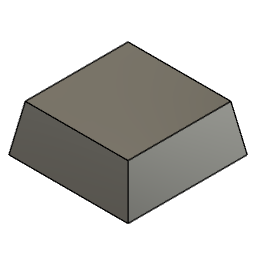
Keycap (Autodesk Fusion 360 design; units mm, degrees)
Autodesk Fusion 360 part; units mm, degrees
sketch "Sketch1" plane through (0, 0, 0) normal (0, 0, 1) x (1, 0, 0)
  line L0 (0, 0) -> (18, 0)
  line L1 (0, 0) -> (0, 7) construction
  line L2 (0, 7) -> (19.3695, 7) construction
  line L3 (18, 0) -> (18, 8.9919) construction
  line L4 (0, 0) -> (1.2343, 7)
  line L5 (0, 0) -> (7.108, 0) construction
  line L6 (18, 0) -> (16.7657, 7)
  line L7 (18, 0) -> (25.108, 0) construction
  line L8 (1.2343, 7) -> (16.7657, 7)
  dimension "d1" = 18
  dimension "d2" = 7
  dimension "d3" = 80
  dimension "d4" = 100
  constraint coincident L0.start L1.start
  constraint horizontal L0
  constraint perpendicular L0 L1
  constraint perpendicular L1 L2
  constraint perpendicular L2 L3
  constraint horizontal L5
  constraint coincident L2 L4.end
  constraint horizontal L7
  constraint coincident L2 L6.end
  measures "d1" distance of L0.start L0.end
  measures "d2" distance of L0.start L1.end
  measures "d3" angle of L4 L5
  measures "d4" angle of L6 L7
extrude "Extrude1" add sketch "Sketch1" along normal blind 18 makes body 1
sketch "Sketch2" plane through (0, 0, 0) normal (1, 0, 0) x (0, 0, -1)
  line L0 (0, 7) -> (0, 0)
  line L1 (0, 0) -> (-18, 0)
  line L2 (-18, 0) -> (-18, 7)
  line L3 (-18, 7) -> (0, 7)
  line L4 (0, 0) -> (-1.2343, 7)
  line L5 (0, 0) -> (7.108, 0) construction
  line L6 (-18, 0) -> (-16.7657, 7)
  line L7 (-18, 0) -> (-10.892, 0) construction
  line L8 (-16.7657, 7) -> (-18, 7)
  line L9 (-18, 7) -> (-18, 0)
  line L10 (-1.2343, 7) -> (0, 7)
  line L11 (0, 7) -> (0, 0)
  dimension "d7" = 100
  dimension "d8" = 80
  constraint horizontal L5
  constraint coincident L0.end L1.start
  constraint coincident L3 L4.end
  constraint horizontal L7
  constraint coincident L1.end L2.start
  constraint coincident L3 L6.end
  constraint coincident L2.end L3.start
  constraint coincident L0.start L3.end
  measures "d7" angle of L4 L5
  measures "d8" angle of L6 L7
extrude "Extrude2" cut sketch "Sketch2" along normal blind 25.5 contours L0 L3 L4 L10 L11 | L2 L3 L6 L8 L9 bodies 1
shell "Shell1" thickness 1.5 removed faces 1 at (6, 0, 6) on bodies 1
sketch "Sketch3" plane through (0, 0, 0) normal (0, 0, 1) x (1, 0, 0)
  line L0 (0, 0) -> (0, 6.75)
  line L1 (3.1, 6.75) -> (3.4, 0)
  line L2 (3.1, 6.75) -> (4.6, 6.75)
  line L3 (3.4, 0) -> (4.9, 0)
  line L4 (4.6, 6.75) -> (4.9, 0)
  dimension "d12" = 6.75
  dimension "d13" = 3.4
  dimension "d14" = 3.1
  dimension "d15" = 4.6
  dimension "d16" = 4.9
  constraint coincident L0.start origin
  constraint vertical L0
  constraint perpendicular L0 L2
  constraint perpendicular L0 L3
  measures "d12" distance of L0.start L0.end
  measures "d13" distance of L0.start L1.end
  measures "d14" distance of L0.end L1.start
  measures "d15" distance of L0.end L2.end
  measures "d16" distance of L0.start L3.end
revolve "Revolve1" add sketch "Sketch3" angle 360 about axis through (0, 0, 0) along (0, 1, 0) separate body makes body 2
move_body "Move1" bodies 2 to x (1, 0, 0) y (0, 1, 0) z (0, 0, 1) at (45, 0, 0)
move_body "Move2" bodies 2 to x (1, 0, 0) y (0, 1, 0) z (0, 0, 1) at (-16, 0, 0)
move_face "OffsetFaces1" offset -1.5 1 faces at (33.0829, 6.75, 0.2285) on bodies 2
move_body "Move3" bodies 2 to x (1, 0, 0) y (0, 1, 0) z (0, 0, 1) at (-20, 0, -9)
move_body "Move4" bodies 2 to x (1, 0, 0) y (0, 1, 0) z (0, 0, 1) at (0, 0, 18)
move_body "Move5" bodies 2 to x (1, 0, 0) y (0, 1, 0) z (0, 0, 1) at (0, 0.3, 0)
combine "Combine1" operation add target body 2 tool bodies 1
fillet "Fillet2" radius 1 1 edges at (4.6471, 5.5, 7.3117) on bodies 2
fillet "Fillet1" [suppressed]
